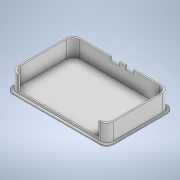
# Autodesk Inventor part: víko
Saved by Autodesk Inventor 2021 (Build 250183000, 183)
## iProperties
Created: 2020-12-03
Part Number: víko
Material: Všeobecné
Document SubType Name: Modeling
Designer: Adam
Density: 1 g/cm^3
Appearance: Výchozí
Author: Adam
Autodesk Inventor part; units mm, degrees
ref_plane "YZ Plane" through (0, 0, 0) normal (1, 0, 0) x (0, 1, 0)
ref_plane "XZ Plane" through (0, 0, 0) normal (0, 1, 0) x (-1, 0, 0)
ref_plane "XY Plane" through (0, 0, 0) normal (0, 0, 1) x (1, 0, 0)
sketch "Náčrt1" plane through (0, 0, 0) normal (0, 1, 0) x (-1, 0, 0)
  line L0 (0, 0) -> (-150, 0)
  line L1 (-150, 0) -> (-150, -100)
  line L2 (-150, -100) -> (0, -100)
  line L3 (0, -100) -> (0, 0)
  dimension "d0" = 150
  dimension "d1" = 100
  constraints: 8 end point, 2 parallel, 1 horizontal, 1 perpendicular
  measures "d0" distance of L2.end L1.end
  measures "d1" distance of L1.end L0.end
extrude "Vysunutí1" add sketch "Náčrt1" along normal blind 1.5
fillet "Zaoblení1" radius 10 4 edges at (150, 0.75, -100) (150, 0.75, 0) (0, 0.75, 0) (0, 0.75, -100)
sketch "Náčrt3" plane through (0, 1.5, 0) normal (0, 1, 0) x (1, 0, 0)
  line L0 (3.5, 96.5) -> (146.5, 96.5)
  line L1 (146.5, 96.5) -> (146.5, 3.5)
  line L2 (146.5, 3.5) -> (3.5, 3.5)
  line L3 (3.5, 3.5) -> (3.5, 96.5)
  line L4 (0, 90) -> (0, 10) projected
  line L5 (10, 0) -> (140, 0) projected
  point P0 (0, 0)
  dimension "d11" = 3.5
  dimension "d12" = 3.5
  dimension "d13" = 93
  dimension "d14" = 143
  constraints: 8 end point, 2 parallel, 1 horizontal, 1 perpendicular
  measures "d11" distance between parallel lines of L4 L3
  measures "d12" distance between parallel lines of L5 L2
  measures "d13" distance of L0.end L1.end
  measures "d14" distance of L0.start L0.end
extrude "Vysunutí3" add sketch "Náčrt3" along normal blind 25
sketch "Náčrt4" plane through (0, 26.5, 0) normal (0, 1, 0) x (1, 0, 0)
  line L0 (3.5, 96.5) -> (3.5, 3.5) projected
  line L1 (5.5, 94.5) -> (144.5, 94.5)
  line L2 (144.5, 94.5) -> (144.5, 5.5)
  line L3 (144.5, 5.5) -> (5.5, 5.5)
  line L4 (5.5, 5.5) -> (5.5, 94.5)
  line L5 (3.5, 3.5) -> (146.5, 3.5) projected
  point P0 (0, 0)
  point P1 (3.5, 13.5)
  point P2 (13.5, 3.5)
  point P3 (136.5, 3.5)
  dimension "d19" = 2
  dimension "d20" = 2
  dimension "d21" = 139
  dimension "d22" = 89
  constraints: 8 end point, 2 parallel, 1 horizontal, 1 perpendicular
  measures "d19" distance between parallel lines of L0 L4
  measures "d20" distance between parallel lines of L5 L3
  measures "d21" distance of L1.start L1.end
  measures "d22" distance of L1.end L2.end
extrude "Vysunutí4" cut sketch "Náčrt4" against normal blind 25
fillet "Zaoblení3" radius 10 8 edges at (144.5, 14, -94.5) (5.5, 14, -94.5) (5.5, 14, -5.5) (144.5, 14, -5.5) (3.5, 14, -96.5) (3.5, 14, -3.5) (146.5, 14, -96.5) (146.5, 14, -3.5)
sketch "Náčrt5" plane through (13.5, 1.5, -3.5) normal (0, 0, 1) x (1, 0, 0)
  line L0 (121, 25) -> (2, 25) projected
  line L1 (133, 0) -> (133, 25) projected
  line L2 (-10, 25) -> (-10, 0) projected
  line L3 (121, 0) -> (121, 25) projected
  line L4 (2, 25) -> (2, 0) projected
  line L5 (121, 3) -> (2, 3)
  line L6 (2, 3) -> (2, 25)
  line L7 (2, 25) -> (121, 25)
  line L8 (121, 25) -> (121, 3)
  point P0 (-13.5, -1.5)
  constraints: 8 end point, 2 parallel, 1 horizontal, 1 perpendicular, 1 point on line
extrude "Vysunutí5" cut sketch "Náčrt5" against normal blind 2
sketch "Náčrt6" plane through (136.5, 1.5, -96.5) normal (0, 0, -1) x (-1, 0, 0)
  line L0 (121, 25) -> (2, 25) projected
  line L1 (76, 25) -> (62, 25)
  line L2 (62, 25) -> (62, 20)
  line L3 (62, 20) -> (76, 20)
  line L4 (76, 20) -> (76, 25)
  line L5 (53, 25) -> (41, 25)
  line L6 (41, 25) -> (41, 20)
  line L7 (41, 20) -> (53, 20)
  line L8 (53, 20) -> (53, 25)
  line L9 (123, 25) -> (123, 0) projected
  line L10 (0, 0) -> (0, 25) projected
  point P0 (136.5, -1.5)
  point P1 (41, 25)
  dimension "d30" = 47
  dimension "d31" = 61
  dimension "d32" = 41
  dimension "d33" = 53
  dimension "d34" = 5
  constraints: 16 end point, 4 parallel, 3 point on line, 2 horizontal, 2 perpendicular
  measures "d30" distance between parallel lines of L4 L9
  measures "d31" distance between parallel lines of L2 L9
  measures "d32" distance between parallel lines of L10 L6
  measures "d33" distance between parallel lines of L8 L10
  measures "d34" distance between parallel lines of L0 L3
extrude "Vysunutí6" cut sketch "Náčrt6" against normal blind 2
